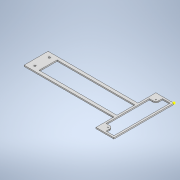
# Autodesk Inventor part: druga czesc
Saved by Autodesk Inventor 2020 (Build 240168000, 168)
## iProperties
Created: 2023-03-09
Part Number: druga czesc
Material: Generic
Document SubType Name: Modeling
Designer: aniela
Density: 1 g/cm^3
Appearance: Default
Author: aniela
Autodesk Inventor part; units mm, degrees
ref_plane "YZ Plane" through (0, 0, 0) normal (1, 0, 0) x (0, 1, 0)
ref_plane "XZ Plane" through (0, 0, 0) normal (0, 1, 0) x (-1, 0, 0)
ref_plane "XY Plane" through (0, 0, 0) normal (0, 0, 1) x (1, 0, 0)
sketch "Sketch1" plane through (0, 0, 0) normal (0, 1, 0) x (-1, 0, 0)
  line L0 (0, 0) -> (30, 0)
  line L1 (30, 0) -> (30, 100)
  line L2 (30, 100) -> (0, 100)
  line L3 (0, 100) -> (0, 0)
  circle A0 centre (20, 90) radius 0.75
  circle A1 centre (20, 10) radius 0.75
  line L4 (3, 97) -> (3, 3)
  line L5 (30, 100) -> (16, 100)
  line L6 (16, 100) -> (16, 91)
  line L7 (21, 86) -> (30, 86)
  line L8 (30, 86) -> (30, 100)
  line L9 (30, 0) -> (16, 0)
  line L10 (16, 0) -> (16, 9)
  line L11 (21, 14) -> (30, 14)
  line L12 (30, 14) -> (30, 0)
  line L13 (27, 86) -> (27, 14)
  line L14 (3, 97) -> (16, 97)
  line L15 (3, 3) -> (16, 3)
  arc A2 (16, 91) -> (21, 86) centre (21, 91) ccw
  arc A3 (21, 14) -> (16, 9) centre (21, 9) ccw
  point P0 (16, 86)
  point P1 (16, 14)
  dimension "d0" = 30
  dimension "d1" = 100
  dimension "d4" = 94
  dimension "d5" = 14
  dimension "d6" = 14
  dimension "d7" = 14
  dimension "d10" = 5
  constraints: 32 end point, 9 point on line, 6 parallel, 6 perpendicular, 4 centre point, 4 point on circle, 4 tangent, 3 coincident, 3 horizontal, 1 equal radius
  measures "d0" distance of L2.end L1.end
  measures "d1" distance of L1.end L0.end
  measures "d4" distance of L4.end L4.start
  measures "d5" distance of L7.end point (16, 86)
  measures "d6" distance of point (16, 86) L5.end
  measures "d7" distance of L9.end point (16, 14)
  measures "d10" radius of A2
extrude "Extrusion1" add sketch "Sketch1" along normal blind 2 contours L3 L2 L6 L14 L4 L15 L10 L0 | L10 A3 L11 L1 L0 | L2 L1 L7 A2 L6 | L11 L13 L7 L1
sketch "Sketch2" plane through (0, 2, 0) normal (0, 1, 0) x (1, 0, 0)
  line L0 (-30, 0) -> (-30, -100) projected
  line L1 (-30, -30) -> (-180, -30)
  line L2 (-180, -30) -> (-180, -70)
  line L3 (-180, -70) -> (-30, -70)
  line L4 (-30, -35) -> (-160, -35)
  line L5 (-160, -35) -> (-160, -65)
  line L6 (-160, -65) -> (-30, -65)
  circle A0 centre (-170, -38) radius 1.5
  circle A1 centre (-170, -62) radius 1.5
  point P0 (0, 0)
  point P1 (-180, -38)
  point P2 (-180, -62)
  point P3 (-180, -62)
  dimension "d11" = 130
  dimension "d12" = 30
  dimension "d13" = 3
  dimension "d14" = 3
  constraints: 12 end point, 6 coincident, 5 perpendicular, 5 point on line, 2 centre point, 1 horizontal
  measures "d11" distance of L4.start L4.end
  measures "d12" distance of L4.end L5.end
  measures "d13" diameter of A0
  measures "d14" diameter of A1
extrude "Extrusion2" add sketch "Sketch2" along normal blind 2 from surface at -2 contours L0 L4 L5 L6 L3 L2 L1
sketch "Sketch5" plane through (0, 2, 0) normal (0, 1, 0) x (1, 0, 0)
  point P0 (0, 0)
body "Solid1"
